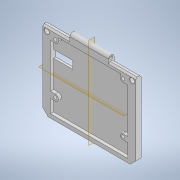
# Autodesk Inventor part: LCD Mount 2
Saved by Autodesk Inventor 2022 (Build 260153000, 153)
## iProperties
Created: 2022-04-02
Part Number: LCD Mount 2
Material: Generic
Document SubType Name: Modeling
Designer: Nick
Density: 1 g/cm^3
Appearance: Default
Author: Nick
Autodesk Inventor part; units mm, degrees
ref_plane "YZ Plane" through (0, 0, 0) normal (1, 0, 0) x (0, 1, 0)
ref_plane "XZ Plane" through (0, 0, 0) normal (0, 1, 0) x (-1, 0, 0)
ref_plane "XY Plane" through (0, 0, 0) normal (0, 0, 1) x (1, 0, 0)
sketch "Sketch1" plane through (0, 0, 0) normal (0, 0, 1) x (1, 0, 0)
  line L0 (0, 100) -> (120, 100)
  line L1 (120, 100) -> (120, 0)
  line L2 (120, 0) -> (0, 0)
  line L3 (0, 0) -> (0, 100)
  line L4 (35, 100) -> (85, 100)
  line L5 (85, 100) -> (85, 107)
  line L6 (85, 107) -> (35, 107)
  line L7 (35, 107) -> (35, 100)
  point P0 (60, 100)
  dimension "d0" = 120
  dimension "d1" = 50
  dimension "d2" = 7
  dimension "d3" = 100
  constraints: 16 end point, 4 parallel, 2 horizontal, 2 midpoint, 2 perpendicular, 1 coincident, 1 point on line
  measures "d0" distance of L1.end L2.end
  measures "d1" distance of L5.end L6.end
  measures "d2" distance of L6.end L4.start
  measures "d3" distance of L2.end L0.start
extrude "Extrusion1" add sketch "Sketch1" along normal blind 7
fillet "Fillet1" radius 3.5 2 edges at (60, 107, 7) (60, 107, 0)
sketch "Sketch2" plane through (85, 100, 7) normal (1, 0, 0) x (0, 0, -1)
  arc A0 (7, 3.5) -> (0, 3.5) centre (3.5, 3.5) ccw projected
  line L0 (0, 0) -> (0, 3.5) projected
  line L1 (7, 0) -> (0, 0) projected
  line L2 (7, 0) -> (7, 3.5) projected
  circle A1 centre (3.5, 3.5) radius 1
  point P0 (7, -100)
  dimension "d7" = 2
  constraints: 1 centre point, 1 coincident
  measures "d7" diameter of A1
extrude "Extrusion2" cut sketch "Sketch2" against normal through all contours A1
ref_plane "Work Plane1" through (60, 0, 0) normal (1, 0, 0) x (0, 0, -1)
ref_plane "Work Plane2" through (0, 50, 0) normal (0, 1, 0) x (1, 0, 0)
chamfer "Chamfer1" distance 2 angle 45 4 edges at (17.5, 100, 7) (17.5, 100, 0) (102.5, 100, 0) (102.5, 100, 7)
sketch "Sketch3" plane through (0, 0, 7) normal (0, 0, 1) x (1, 0, 0)
  circle A0 centre (115, 94.5058) radius 3 projected
  circle A1 centre (5, 94.5058) radius 3 projected
  point P0 (0, 0)
extrude "Extrusion3" cut sketch "Sketch3" against normal blind 6
chamfer "Chamfer2" distance 0.5 angle 45 2 edges at (112, 94.5058, 7) (2, 94.5058, 7)
sketch "Sketch4" plane through (0, 0, 7) normal (0, 0, 1) x (1, 0, 0)
  line L0 (10, 95) -> (110, 95)
  line L1 (110, 95) -> (110, 5)
  line L2 (110, 5) -> (10, 5)
  line L3 (10, 5) -> (10, 95)
  line L4 (35, 100) -> (0, 100) projected
  line L5 (0, 98) -> (0, 0) projected
  line L6 (120, 0) -> (120, 98) projected
  line L7 (0, 0) -> (120, 0) projected
  line L8 (16.225, 91) -> (103.775, 91) construction
  line L9 (103.775, 91) -> (103.775, 26.1) construction
  line L10 (103.775, 26.1) -> (16.225, 26.1) construction
  line L11 (16.225, 26.1) -> (16.225, 91) construction
  circle A0 centre (16.225, 91) radius 4
  line L12 (20.225, 91) -> (20.225, 95)
  line L13 (16.225, 87) -> (10, 87)
  circle A1 centre (16.225, 26.1) radius 4
  line L14 (16.225, 30.1) -> (10, 30.1)
  line L15 (16.225, 22.1) -> (10, 22.1)
  circle A2 centre (103.775, 91) radius 4
  circle A3 centre (103.775, 26.1) radius 3.5
  line L16 (103.775, 29.6) -> (110, 29.6)
  line L17 (103.775, 22.6) -> (110, 22.6)
  line L18 (99.775, 91) -> (99.775, 95)
  line L19 (103.775, 87) -> (110, 87)
  point P0 (60, 91)
  point P1 (60, 95)
  dimension "d18" = 5
  dimension "d19" = 10
  dimension "d20" = 10
  dimension "d21" = 5
  dimension "d24" = 87.55
  dimension "d25" = 64.9
  dimension "d26" = 4
  dimension "d27" = 8
  dimension "d28" = 8
  dimension "d29" = 8
  dimension "d30" = 7
  constraints: 32 end point, 10 perpendicular, 8 point on circle, 8 point on line, 8 tangent, 4 centre point, 4 coincident, 4 parallel, 2 horizontal, 2 midpoint, 1 vertical alignment
  measures "d18" distance between parallel lines of L0 L4
  measures "d19" distance between parallel lines of L5 L3
  measures "d20" distance between parallel lines of L6 L1
  measures "d21" distance between parallel lines of L7 L2
  measures "d24" distance of L9.end L10.end
  measures "d25" distance of L8.end L9.end
  measures "d26" distance from line of L0 L8.start
  measures "d27" diameter of A0
  measures "d28" diameter of A1
  measures "d29" diameter of A2
  measures "d30" diameter of A3
extrude "Extrusion4" cut sketch "Sketch4" against normal blind 4 contours L0 L18 A2 L19 L1 L16 A3 L17 L2 L3 L15 A1 L14 L13 A0 L12
sketch "Sketch5" plane through (0, 0, 7) normal (0, 0, 1) x (1, 0, 0)
  line L0 (103.775, 22.6) -> (110, 22.6) projected
  line L1 (110, 22.6) -> (110, 5) projected
  line L2 (110, 5) -> (10, 5) projected
  line L3 (10, 5) -> (10, 22.1) projected
  line L4 (10, 22.1) -> (16.225, 22.1) projected
  arc A0 (16.225, 22.1) -> (16.225, 30.1) centre (16.225, 26.1) ccw projected
  line L5 (16.225, 30.1) -> (10, 30.1) projected
  line L6 (10, 30.1) -> (10, 87) projected
  line L7 (10, 87) -> (16.225, 87) projected
  arc A1 (16.225, 87) -> (20.225, 91) centre (16.225, 91) ccw projected
  line L8 (20.225, 91) -> (20.225, 95) projected
  line L9 (20.225, 95) -> (99.775, 95) projected
  line L10 (99.775, 95) -> (99.775, 91) projected
  arc A2 (99.775, 91) -> (103.775, 87) centre (103.775, 91) ccw projected
  line L11 (103.775, 87) -> (110, 87) projected
  line L12 (110, 87) -> (110, 29.6) projected
  line L13 (110, 29.6) -> (103.775, 29.6) projected
  arc A3 (103.775, 29.6) -> (103.775, 22.6) centre (103.775, 26.1) ccw projected
  arc A4 (4.798, 98) -> (5.202, 98) centre (5, 94.5058) ccw projected
  line L14 (0, 98) -> (4.798, 98) projected
  line L15 (0, 98) -> (0, 0) projected
  line L16 (0, 0) -> (120, 0) projected
  line L17 (120, 0) -> (120, 98) projected
  line L18 (115.202, 98) -> (120, 98) projected
  arc A5 (114.798, 98) -> (115.202, 98) centre (115, 94.5058) ccw projected
  line L19 (85, 98) -> (114.798, 98) projected
  line L20 (85, 98) -> (85, 103.5) projected
  line L21 (35, 103.5) -> (85, 103.5) projected
  line L22 (35, 103.5) -> (35, 98) projected
  line L23 (5.202, 98) -> (35, 98) projected
hole "Hole1" at (16.225, 91, 7) at (16.225, 26.1, 7) at (103.775, 26.1, 7) at (103.775, 91, 7) direction (0, 0, -1) diameter 4 end through all
sketch "Sketch6" plane through (0, 0, 3) normal (0, 0, 1) x (1, 0, 0)
  line L0 (10, 30.1) -> (10, 87) projected
  line L1 (10, 75) -> (35, 75)
  line L2 (35, 75) -> (35, 65)
  line L3 (35, 65) -> (10, 65)
  line L4 (10, 65) -> (10, 75)
  line L5 (20.225, 95) -> (99.775, 95) projected
  point P0 (0, 0)
  point P1 (10, 65)
  dimension "d40" = 20
  dimension "d41" = 10
  dimension "d42" = 25
  constraints: 8 end point, 2 parallel, 1 horizontal, 1 perpendicular, 1 point on line
  measures "d40" distance between parallel lines of L5 L1
  measures "d41" distance of L1.end L2.end
  measures "d42" distance of L2.end L3.end
extrude "Extrusion5" cut sketch "Sketch6" against normal through all
chamfer "Chamfer3" distance 7 angle 45 2 edges at (120, 0, 3.5) (0, 0, 3.5)
chamfer "Chamfer4" distance 1 angle 45 2 edges at (35, 103.5, 4.5) (85, 103.5, 4.5)
body "Solid1"
